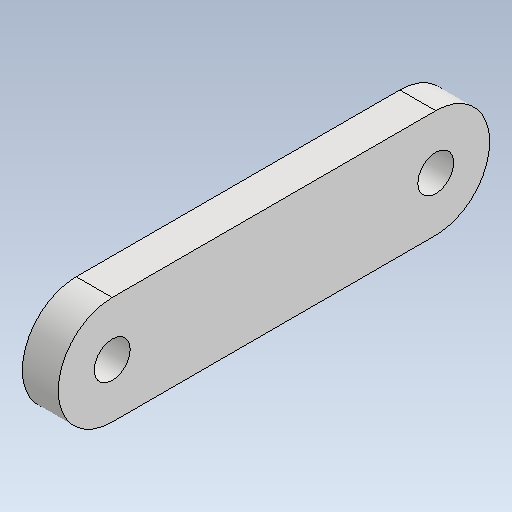
# Autodesk Inventor part: scissor-link-upper
Saved by Autodesk Inventor 2025 (Build 290162000, 162)
## iProperties
Created: 2025-08-20
Part Number: scissor-link-upper
Material: Generic
Document SubType Name: Modeling
Designer: HP
Density: 1 g/cm^3
Appearance: Default
Author: HP
Autodesk Inventor part; units mm, degrees
ref_plane "YZ Plane" through (0, 0, 0) normal (1, 0, 0) x (0, 1, 0)
ref_plane "XZ Plane" through (0, 0, 0) normal (0, 1, 0) x (-1, 0, 0)
ref_plane "XY Plane" through (0, 0, 0) normal (0, 0, 1) x (1, 0, 0)
sketch "Sketch1" plane through (0, 0, 0) normal (1, 0, 0) x (0, 1, 0)
  line L0 (-7.5, 22.5) -> (7.5, 22.5)
  line L1 (7.5, 22.5) -> (7.5, -22.5)
  line L2 (7.5, -22.5) -> (-7.5, -22.5)
  line L3 (-7.5, -22.5) -> (-7.5, 22.5)
  line L4 (-7.5, 22.5) -> (7.5, -22.5) construction
  line L5 (7.5, 22.5) -> (-7.5, -22.5) construction
  circle A0 centre (0, 22.5) radius 7.5
  circle A1 centre (0, -22.5) radius 7.5
  circle A2 centre (0, -22.5) radius 2.5
  circle A3 centre (0, 22.5) radius 2.5
  point P0 (0, 0)
  point P1 (-7.5, 22.5)
  point P2 (-7.5, -22.5)
  dimension "d0" = 15
  dimension "d1" = 5
  dimension "d2" = 5
  dimension "d3" = 45
  constraints: 12 end point, 4 midpoint, 2 centre point, 2 coincident, 2 parallel, 1 horizontal, 1 perpendicular, 6 other
  measures "d0" distance between parallel lines of L3 L1
  measures "d1" diameter of A2
  measures "d2" diameter of A3
  measures "d3" distance between parallel lines of L2 L0
extrude "Extrusion1" add sketch "Sketch1" along normal blind 5 contours A3 L0 A0 | L0 A0 A3 | L1 A1 L3 A0 | A1 L2 A2 | L2 A2 A1
body "Solid1"
